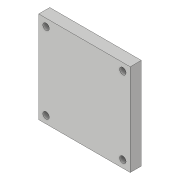
# Autodesk Inventor part: Modulo
Saved by Autodesk Inventor 2017 (Build 210142000, 142)
## iProperties
Created: 2017-06-21
Part Number: Modulo
Material: Generic
Document SubType Name: Modeling
Designer: Butri
Density: 1 g/cm^3
Appearance: Default
Author: Butri
Autodesk Inventor part; units mm, degrees
ref_plane "YZ Plane" through (0, 0, 0) normal (1, 0, 0) x (0, 1, 0)
ref_plane "XZ Plane" through (0, 0, 0) normal (0, 1, 0) x (-1, 0, 0)
ref_plane "XY Plane" through (0, 0, 0) normal (0, 0, 1) x (1, 0, 0)
sketch "Sketch1" plane through (0, 0, 0) normal (0, 1, 0) x (-1, 0, 0)
  line L0 (24.75, -24.75) -> (-24.75, -24.75)
  line L1 (-24.75, -24.75) -> (-24.75, 24.75)
  line L2 (-24.75, 24.75) -> (24.75, 24.75)
  line L3 (24.75, 24.75) -> (24.75, -24.75)
  line L4 (24.75, -24.75) -> (-24.75, 24.75) construction
  line L5 (-24.75, -24.75) -> (24.75, 24.75) construction
  circle A0 centre (20.75, 20.75) radius 1.75
  circle A1 centre (20.75, -20.75) radius 1.75
  circle A2 centre (-20.75, 20.75) radius 1.75
  circle A3 centre (-20.75, -20.75) radius 1.75
  point P0 (0, 0)
  dimension "d0" = 49.5
  dimension "d1" = 49.5
  dimension "d2" = 3.5
  dimension "d3" = 4
  dimension "d4" = 3.5
  dimension "d5" = 4
  dimension "d6" = 3.5
  dimension "d7" = 3.5
  dimension "d8" = 4
  dimension "d14" = 4
  constraints: 12 end point, 4 centre point, 4 point on line, 2 midpoint, 2 parallel, 1 horizontal, 1 perpendicular
  measures "d0" distance of L1.end L2.end
  measures "d1" distance of L0.end L1.end
  measures "d2" diameter of A0
  measures "d3" distance from line of L2 A0.centre
  measures "d4" diameter of A1
  measures "d5" distance from line of L0 A1.centre
  measures "d6" diameter of A2
  measures "d7" diameter of A3
  measures "d8" distance from line of L1 A3.centre
  measures "d14" distance from line of L1 A2.centre
extrude "Extrusion1" add sketch "Sketch1" along normal blind 6
chamfer "Chamfer1" distance 2 angle 45 4 edges at (-19, 6, 20.75) (-19, 6, -20.75) (22.5, 6, 20.75) (22.5, 6, -20.75)
equation "\"d1\" = d0"
equation "\"d4\" = d2"
equation "\"d5\" = d3"
equation "\"d6\" = d2"
equation "\"d7\" = d2"
equation "\"d8\" = d3"
equation "\"d14\" = d3"
body "Solid1"
